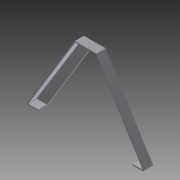
# Autodesk Inventor part: 8 ball lift frame
Saved by Autodesk Inventor 2012 (Build 160160000, 160)
## iProperties
Created: 2013-10-11
Part Number: 8 ball lift frame
Material: Default
Document SubType Name: Modeling
Designer: Bryce
Density: 1 g/cm^3
Author: Bryce
Autodesk Inventor part; units mm, degrees
ref_plane "YZ Plane" through (0, 0, 0) normal (1, 0, 0) x (0, 1, 0)
ref_plane "XZ Plane" through (0, 0, 0) normal (0, 1, 0) x (-1, 0, 0)
ref_plane "XY Plane" through (0, 0, 0) normal (0, 0, 1) x (1, 0, 0)
sketch "Sketch1" plane through (0, 0, 0) normal (0, 0, 1) x (1, 0, 0)
  line L0 (0, 0) -> (33.5477, 0)
  line L1 (136.525, 215.9) -> (193.675, 215.9)
  line L2 (136.525, 215.9) -> (6.6569, 4.7625)
  line L3 (193.675, 215.9) -> (324.5196, 3.175)
  line L4 (330.2, 0) -> (195.4496, 219.075)
  line L5 (195.4496, 219.075) -> (134.7504, 219.075)
  line L6 (134.7504, 219.075) -> (0, 0)
  line L7 (33.5477, 3.175) -> (33.5477, 0)
  line L8 (324.5196, 3.175) -> (296.6523, 3.175)
  line L9 (296.6523, 3.175) -> (296.6523, 0)
  line L10 (6.6569, 4.7625) -> (36.4771, 4.7625)
  line L11 (36.4771, 4.7625) -> (164.3062, 212.5851)
  line L12 (165.8937, 212.5851) -> (293.7229, 4.7625)
  line L13 (293.7229, 4.7625) -> (323.5431, 4.7625)
  line L14 (135.5485, 214.3125) -> (164.3062, 214.3125)
  line L15 (164.3062, 214.3125) -> (164.3062, 212.5851)
  line L16 (165.8937, 212.5851) -> (165.8937, 214.3125)
  line L17 (165.8937, 214.3125) -> (194.6515, 214.3125)
  line L18 (296.6523, 0) -> (330.2, 0)
  line L19 (33.5477, 0) -> (296.6523, 0) construction
  line L20 (6.6569, 4.7625) -> (5.6804, 3.175)
  line L21 (33.5477, 3.175) -> (5.6804, 3.175)
  dimension "d0" = 330.2
  dimension "d1" = 57.15
  dimension "d5" = 3.175
  dimension "d6" = 215.9
  dimension "d30" = 58.405
  dimension "d31" = 3.175
  dimension "d34" = 25.4
  dimension "d35" = 25.4
  dimension "d36" = 1.5875
  dimension "d37" = 1.5875
  dimension "d39" = 1.5875
  dimension "d40" = 58.405
  dimension "d41" = 3.175
  dimension "d42" = 1.5875
  constraints: 44 end point, 15 parallel, 7 perpendicular, 5 point on line, 3 horizontal, 1 horizontal alignment, 1 other
  measures "d0" distance of L0.start L4.start
  measures "d1" distance of L1.start L1.end
  measures "d5" distance between parallel lines of L5 L1
  measures "d6" distance between parallel lines of L0 L1
  measures "d30" angle of L0 L2
  measures "d31" distance of L7.start L0.end
  measures "d34" distance between parallel lines of L11 L2
  measures "d35" distance between parallel lines of L12 L3
  measures "d36" distance between parallel lines of L16 L15
  measures "d37" distance between parallel lines of L1 L14
  measures "d39" distance between parallel lines of L8 L13
  measures "d40" angle of L18 L3
  measures "d41" distance between parallel lines of L6 L2
  measures "d42" distance between parallel lines of L21 L10
extrude "Extrusion1" add sketch "Sketch1" along normal blind 25.4 contours L6 L5 L4 L18 L9 L8 L3 L1 L2 L20 L21 L7 L0
extrude "Extrusion2" add sketch "Sketch1" along normal blind 3.175
fillet "Fillet1" radius 0.7937 8 edges at (5.6804, 3.175, 12.7) (324.5196, 3.175, 12.7) (136.525, 215.9, 12.7) (193.675, 215.9, 12.7) (194.6515, 214.3125, 1.5875) (135.5485, 214.3125, 1.5875) (323.5431, 4.7625, 1.5875) (6.6569, 4.7625, 1.5875)
fillet "Fillet2" radius 3.175 4 edges at (134.7504, 219.075, 12.7) (195.4496, 219.075, 12.7) (330.2, 0, 12.7) (0, 0, 12.7)
equation "\"d5\" = d4"
equation "\"d30\" = d40"
equation "\"d31\" = d5"
equation "\"d36\" = 0.5 * d5"
equation "\"d37\" = d36"
equation "\"d39\" = d38"
equation "\"d42\" = d37"
equation "\"d38\" = d37"
equation "\"d4\" = 3.175"
body "Solid1"
